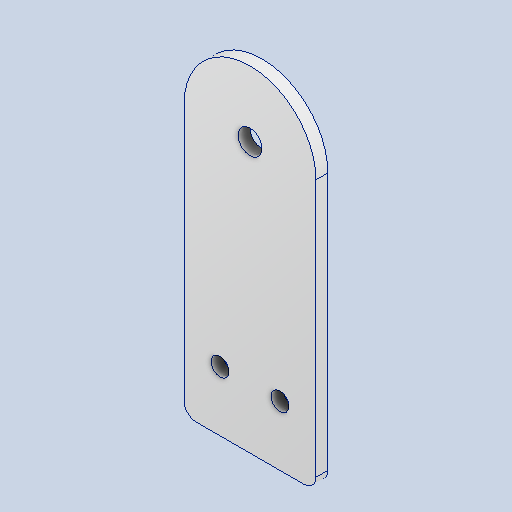
# Autodesk Inventor part: dribl-v3-Plate-17
Saved by Autodesk Inventor 2025.2 (Build 292293000, 293)
## iProperties
Created: 2025-04-12
Part Number: dribl-v3-Plate-17
Material: アルミニウム 6061
Document SubType Name: Modeling
Designer: haruy
Density: 2.7 g/cm^3
Appearance: アルミニウム - フラット
Author: haruy
Autodesk Inventor part; units mm, degrees
ref_plane "YZ Plane" through (0, 0, 0) normal (1, 0, 0) x (0, 1, 0)
ref_plane "XZ Plane" through (0, 0, 0) normal (0, 1, 0) x (-1, 0, 0)
ref_plane "XY Plane" through (0, 0, 0) normal (0, 0, 1) x (1, 0, 0)
derived "dribl-v3-Sketch-Base.ipt"
sketch "スケッチ5" plane through (-180, -184.3334, -303) normal (0, 0, 1) x (1, 0, 0)
  circle A0 centre (37.42, 41) radius 16 projected
  line L0 (0, -248) -> (0, 1189.5) projected
  line L1 (560, 20) -> (0, 20) projected
  circle A1 centre (10, 10) radius 1.6 projected
  circle A2 centre (30, 10) radius 1.6 projected
  line L2 (0, 0) -> (560, 0) projected
  line L3 (280, 20) -> (280, 0) projected
  circle A3 centre (522.58, 41) radius 16 projected
  circle A4 centre (530, 10) radius 1.6 projected
  circle A5 centre (550, 10) radius 1.6 projected
  circle A6 centre (-10, 10) radius 1.6 projected
  circle A7 centre (-10, -10) radius 1.6 projected
  line L4 (-20, 1189.5) -> (-20, -248) projected
  circle A8 centre (570, 10) radius 1.6 projected
  circle A9 centre (570, -10) radius 1.6 projected
  line L5 (420, 0) -> (420, 20) projected
  line L6 (560, -248) -> (560, 1189.5) projected
  line L7 (415, 20) -> (415, 0) projected
  circle A10 centre (404.9, 46) radius 16 projected
  circle A11 centre (404.9, 46) radius 5.1 projected
  line L8 (404.9, 46) -> (404.9, 0) projected
  line L9 (394.8, 20) -> (394.8, 0) projected
  circle A12 centre (404.9, 66) radius 5.1 projected
  circle A13 centre (404.9, 66) radius 10.1 projected
  line L10 (394.8, 20) -> (394.8, 66) projected
  line L11 (415, 20) -> (415, 66) projected
  line L12 (394.8, 66) -> (415, 66) projected
  line L13 (415, 66) -> (415, 76.1) projected
  line L14 (415, 76.1) -> (394.8, 76.1) projected
  line L15 (394.8, 76.1) -> (394.8, 66) projected
  line L16 (399.8, 46) -> (399.8, 66) projected
  line L17 (410, 66) -> (410, 46) projected
  circle A14 centre (410, 10) radius 1.6 projected
  circle A15 centre (400, 10) radius 1.6 projected
  line L18 (394.8, 0) -> (415, 0) projected
  line L19 (415, 0) -> (415, 20) projected
  line L20 (415, 20) -> (394.8, 20) projected
  line L21 (394.8, 20) -> (394.8, 0) projected
  circle A16 centre (404.9, 41) radius 5.1 projected
  line L22 (399.8, 46) -> (399.8, 41) projected
  line L23 (410, 46) -> (410, 41) projected
  circle A17 centre (371.4, 45) radius 11 projected
  circle A18 centre (371.4, 45) radius 2 projected
  circle A19 centre (37.42, 41) radius 12.5 projected
  circle A20 centre (522.58, 41) radius 12.5 projected
  line L24 (522.58, 53.5) -> (37.42, 53.5) projected
  line L25 (37.42, 28.5) -> (522.58, 28.5) projected
  line L26 (360.4, 45) -> (360.4, 0) projected
  line L27 (382.4, 45) -> (382.4, 0) projected
  circle A21 centre (366.4, 10) radius 1.5 projected
  circle A22 centre (376.4, 10) radius 1.5 projected
  line L28 (449.4, 45) -> (449.4, 0) projected
  line L29 (427.4, 45) -> (427.4, 0) projected
  circle A23 centre (438.4, 45) radius 11 projected
  circle A24 centre (438.4, 45) radius 2 projected
  circle A25 centre (443.4, 10) radius 1.5 projected
  circle A26 centre (433.4, 10) radius 1.5 projected
  point P0 (180, 184.3334)
extrude "押し出し1" add sketch "スケッチ5" along normal blind 2 contours L24 A17 | A17 L24 | L26 A17 L27 L25 | L25 L27 L1 L26 | L1 L27 L2 L26
fillet "フィレット1" radius 2 2 edges at (180.4, -184.3334, -302) (202.4, -184.3334, -302)
